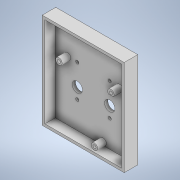
# Autodesk Inventor part: nucleo_din_connector
Saved by Autodesk Inventor 2021 (Build 250183000, 183)
## iProperties
Created: 2020-10-29
Part Number: nucleo_din_connector
Material: Generic
Document SubType Name: Modeling
Designer: Mateusz
Density: 1 g/cm^3
Appearance: Default
Author: Mateusz
Autodesk Inventor part; units mm, degrees
ref_plane "YZ Plane" through (0, 0, 0) normal (1, 0, 0) x (0, 1, 0)
ref_plane "XZ Plane" through (0, 0, 0) normal (0, 1, 0) x (-1, 0, 0)
ref_plane "Work Plane1" through (-41.89, 79.898, 0.7952) normal (0, 0, 1) x (1, 0, 0)
sketch "Sketch1" plane through (-41.89, 79.898, 0.7952) normal (0, 0, 1) x (1, 0, 0)
  circle A0 centre (41.89, -79.898) radius 1.45
  circle A1 centre (8.87, -27.828) radius 1.45
  circle A2 centre (57.13, -29.098) radius 1.45
  arc A3 (66, -80.398) -> (68, -78.398) centre (66, -78.398) ccw projected
  line L0 (66, 0.102) -> (0, 0.102) projected
  line L1 (-2, -1.898) -> (-2, -24.398) projected
  line L2 (-2, 0.102) -> (68, 0.102)
  line L3 (68, 0.102) -> (68, -82.398)
  line L4 (68, -82.398) -> (-2, -82.398)
  line L5 (-2, -82.398) -> (-2, 0.102)
  line L6 (-2, 3.102) -> (-5, 3.102)
  line L7 (68, -85.398) -> (71, -85.398)
  line L8 (-5, 3.102) -> (71, 3.102)
  line L9 (71, 3.102) -> (71, -85.398)
  line L10 (71, -85.398) -> (-5, -85.398)
  line L11 (-5, -85.398) -> (-5, 3.102)
  point P0 (44.5, -82.398)
  point P1 (-2, 3.102)
  point P2 (-2, -24.398)
  point P3 (-2, -1.898)
  point P4 (66, 0.102)
  dimension "d0" = 2.9
  dimension "d1" = 2.9
  dimension "d2" = 2.9
  constraints: 20 end point, 4 parallel, 3 centre point, 2 horizontal, 2 perpendicular
  measures "d0" diameter of A0
  measures "d1" diameter of A1
  measures "d2" diameter of A2
extrude "Extrusion1" add sketch "Sketch1" against normal blind 3 contours L2 L3 L4 L5 L1 L0 | L8 L9 L7 L10 L11 L6
sketch "Sketch2" plane through (-41.89, 79.898, 0.7952) normal (0, 0, 1) x (1, 0, 0)
  circle A0 centre (8.87, -27.828) radius 1.45 projected
  circle A1 centre (8.87, -27.828) radius 3
  circle A2 centre (57.13, -29.098) radius 1.45 projected
  circle A3 centre (57.13, -29.098) radius 3
  circle A4 centre (41.89, -79.898) radius 3
  circle A5 centre (41.89, -79.898) radius 1.45
  dimension "d9" = 6
  dimension "d10" = 6
  dimension "d11" = 6
  constraints: 4 centre point, 4 coincident
  measures "d9" diameter of A1
  measures "d10" diameter of A3
  measures "d11" diameter of A4
extrude "Extrusion2" add sketch "Sketch2" along normal blind 3
sketch "Sketch3" plane through (-41.89, 79.898, 0.7952) normal (0, 0, 1) x (1, 0, 0)
  line L0 (71, -85.398) -> (-5, -85.398) projected
  circle A0 centre (18, -27.898) radius 1.45
  circle A1 centre (48, -27.898) radius 1.45
  circle A2 centre (18, -57.898) radius 1.45
  circle A3 centre (48, -57.898) radius 1.45
  point P0 (41.89, -79.898)
  dimension "d19" = 2.9
  dimension "d20" = 2.9
  dimension "d21" = 2.9
  dimension "d22" = 2.9
  constraints: 4 centre point
  measures "d19" diameter of A0
  measures "d20" diameter of A1
  measures "d21" diameter of A2
  measures "d22" diameter of A3
extrude "Extrusion3" cut sketch "Sketch3" against normal up to surface (3 mm away)
extrude "Extrusion5" add sketch "Sketch1" along normal blind 4.58 contours L8 L9 L7 L10 L11 L6
sketch "Sketch5" plane through (-41.89, 79.898, 5.3752) normal (0, 0, 1) x (1, 0, 0)
  line L0 (-2, 0.102) -> (-2, -82.398) projected
  line L1 (-2, -82.898) -> (68, -82.898)
  line L2 (43.5483, -82.398) -> (68, -82.398) projected
  line L3 (68, -82.898) -> (68.5, -82.898)
  line L4 (68.5, -82.898) -> (68.5, 0.102)
  line L5 (68, -82.398) -> (68, 0.102) projected
  line L6 (68.5, 0.102) -> (68.5, 0.602)
  line L7 (68.5, 0.602) -> (-2, 0.602)
  line L8 (-2, 0.602) -> (-2.5, 0.602)
  line L9 (-2.5, 0.602) -> (-2.5, -82.898)
  line L10 (-2.5, -82.898) -> (-2, -82.898)
  line L11 (-2, -82.398) -> (-2, 0.102) projected
  line L12 (68, -82.398) -> (-2, -82.398) projected
  line L13 (68, 0.102) -> (68, -82.398) projected
  line L14 (-2, 0.102) -> (68, 0.102) projected
  point P0 (41.89, -79.898)
  dimension "d33" = 0.5
  dimension "d34" = 0.5
  dimension "d35" = 0.5
  dimension "d36" = 0.5
  constraints: 16 end point, 4 point on line, 3 perpendicular, 2 parallel
  measures "d33" distance of L0.end L1.start
  measures "d34" distance of L1.end L3.end
  measures "d35" distance of L4.end L6.end
  measures "d36" distance of L7.end L8.end
extrude "Extrusion6" cut sketch "Sketch5" against normal up to surface (4.58 mm away)
sketch "Sketch6" plane through (-41.89, 79.898, 0.7952) normal (0, 0, 1) x (1, 0, 0)
  circle A0 centre (48, -57.898) radius 1.45 projected
  circle A1 centre (18, -57.898) radius 1.45 projected
  circle A2 centre (48, -47.966) radius 4.767
  circle A3 centre (18, -47.966) radius 4.767
  point P0 (41.89, -79.898)
  dimension "d40" = 9.534
  constraints: 2 centre point
  measures "d40" diameter of A2
extrude "Extrusion7" cut sketch "Sketch6" against normal up to surface (3 mm away) contours A2 | A3
sketch "Sketch7" plane through (15.24, 50.8, 3.7952) normal (0, 0, 1) x (1, 0, 0)
  line L0 (-16.8983, -53.3) -> (-13.5817, -53.3) projected
  arc A0 (-13.5817, -53.3) -> (-16.8983, -53.3) centre (-15.24, -50.8) ccw projected
  circle A1 centre (-15.24, -50.8) radius 1.45 projected
  circle A2 centre (-48.26, 1.27) radius 3 projected
  circle A3 centre (-48.26, 1.27) radius 1.45 projected
  circle A4 centre (0, 0) radius 3 projected
  circle A5 centre (0, 0) radius 1.45 projected
  point P0 (-15.24, -50.8)
extrude "Extrusion8" add sketch "Sketch7" along normal blind 5
sketch "Sketch8" plane through (-41.89, 79.898, 5.3752) normal (0, 0, 1) x (1, 0, 0)
  line L0 (68.5, -82.898) -> (-2.5, -82.898) projected
  line L1 (-2.5, -82.898) -> (-2.5, 0.602) projected
  line L2 (-2.5, 0.602) -> (68.5, 0.602) projected
  line L3 (68.5, 0.602) -> (68.5, -82.898) projected
  line L4 (71, 3.102) -> (-5, 3.102) projected
  line L5 (-5, 3.102) -> (-5, -85.398) projected
  line L6 (-5, -85.398) -> (71, -85.398) projected
  line L7 (71, -85.398) -> (71, 3.102) projected
  point P0 (41.89, -79.898)
extrude "Extrusion9" add sketch "Sketch8" along normal blind 5
sketch "Sketch9" plane through (15.24, 50.8, 8.7952) normal (0, 0, 1) x (1, 0, 0)
  circle A0 centre (0, 0) radius 1.45 projected
  circle A1 centre (0, 0) radius 3 projected
  line L0 (0, 0) -> (0, -2)
  line L1 (0, -2) -> (2.2361, -2)
  line L2 (0, -2) -> (-2.2361, -2)
  point P0 (-15.24, -50.8)
  dimension "d47" = 2
  constraints: 6 end point, 2 point on circle, 1 perpendicular, 1 point on line, 1 vertical
  measures "d47" distance of L0.start L0.end
extrude "Extrusion10" cut sketch "Sketch9" against normal up to surface (8 mm away) contours L1 A1 L2 picked at (1.3106, -2.1582)
sketch "Sketch10" plane through (-41.89, 79.898, 0.7952) normal (0, 0, 1) x (1, 0, 0)
  arc A0 (43.5483, -82.398) -> (40.2317, -82.398) centre (41.89, -79.898) ccw projected
  circle A1 centre (41.89, -79.898) radius 3
  circle A2 centre (41.89, -79.898) radius 1.45 projected
  circle A3 centre (41.89, -79.898) radius 1.45
  point P0 (41.89, -79.898)
  point P1 (40.2317, -82.398)
  constraints: 2 centre point, 2 coincident
extrude "Extrusion11" add sketch "Sketch10" along normal up to surface (8 mm away)
body "Solid2044"
